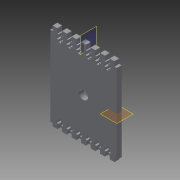
# Autodesk Inventor part: yokeEndBlock
Saved by Autodesk Inventor 2013 (Build 170138000, 138)
## iProperties
Created: 2013-02-24
Part Number: yokeEndBlock
Material: Generic
Document SubType Name: Modeling
Designer: Nano
Density: 1 g/cm^3
d0: 0.250 in
d1: 0.00 deg
d2: 0.250 in
d3: 4.000 ul
d5: 0.500 in
d10: 0.250 in
d11: 0.00 deg
d14: 0.375 in
d21: 0.125 in
d22: 0.600 in
d23: 0.313 in
d24: 0.125 in
d25: 0.375 in
d27: 0.00 deg
d28: 6.000 ul
d30: 0.500 in
Author: Nano
Autodesk Inventor part; units mm, degrees
ref_plane "YZ Plane" through (0, 0, 0) normal (1, 0, 0) x (0, 1, 0)
ref_plane "XZ Plane" through (0, 0, 0) normal (0, 1, 0) x (-1, 0, 0)
ref_plane "XY Plane" through (0, 0, 0) normal (0, 0, 1) x (1, 0, 0)
ref_plane "Work Plane1" through (0, 0, 0) normal (0, 0, 1) x (1, 0, 0)
sketch "Sketch1" plane through (0, 0, 0) normal (0, 0, 1) x (1, 0, 0)
  circle A0 centre (44.45, -59.5313) radius 5.9531
  line L0 (0, 0) -> (0, -116.6812)
  line L1 (0, -116.6812) -> (88.9, -116.6812)
  line L2 (88.9, 0) -> (88.9, -116.6812)
  line L3 (0, 0) -> (88.9, 0)
  dimension "d31" = 11.9062
  dimension "d33" = 116.6813
  constraints: 8 end point, 1 centre point, 1 other
  measures "d31" diameter of A0
  measures "d33" distance of L2.start L1.end
extrude "Extrusion1" add sketch "Sketch1" along normal blind 6.35
sketch "Sketch2" plane through (0, 0, 0) normal (0, 1, 0) x (1, 0, 0)
  line L0 (88.9, 0) -> (0, 0) projected
  line L1 (0, 0) -> (0, -6.35) projected
  line L2 (88.9, -6.35) -> (0, -6.35) projected
  line L3 (88.9, 0) -> (88.9, -6.35) projected
  line L4 (41.275, -6.35) -> (41.275, 0)
  line L5 (41.275, 0) -> (47.625, 0)
  line L6 (47.625, 0) -> (47.625, -6.35)
  line L7 (47.625, -6.35) -> (41.275, -6.35)
  line L8 (41.275, -6.35) -> (47.625, 0) construction
  line L9 (41.275, 0) -> (47.625, -6.35) construction
  line L10 (28.575, -6.35) -> (28.575, 0)
  line L11 (28.575, 0) -> (34.925, 0)
  line L12 (34.925, 0) -> (34.925, -6.35)
  line L13 (34.925, -6.35) -> (28.575, -6.35)
  line L14 (28.575, -6.35) -> (34.925, 0) construction
  line L15 (28.575, 0) -> (34.925, -6.35) construction
  line L16 (15.875, -6.35) -> (15.875, 0)
  line L17 (15.875, 0) -> (22.225, 0)
  line L18 (22.225, 0) -> (22.225, -6.35)
  line L19 (22.225, -6.35) -> (15.875, -6.35)
  line L20 (15.875, -6.35) -> (22.225, 0) construction
  line L21 (15.875, 0) -> (22.225, -6.35) construction
  line L22 (3.175, -6.35) -> (3.175, 0)
  line L23 (3.175, 0) -> (9.525, 0)
  line L24 (9.525, 0) -> (9.525, -6.35)
  line L25 (9.525, -6.35) -> (3.175, -6.35)
  line L26 (3.175, -6.35) -> (9.525, 0) construction
  line L27 (3.175, 0) -> (9.525, -6.35) construction
  line L28 (44.45, 0) -> (44.45, -6.35) construction
  line L29 (60.325, -6.35) -> (60.325, 0)
  line L30 (60.325, 0) -> (53.975, 0)
  line L31 (53.975, 0) -> (53.975, -6.35)
  line L32 (53.975, -6.35) -> (60.325, -6.35)
  line L33 (60.325, -6.35) -> (53.975, 0) construction
  line L34 (60.325, 0) -> (53.975, -6.35) construction
  line L35 (73.025, -6.35) -> (73.025, 0)
  line L36 (73.025, 0) -> (66.675, 0)
  line L37 (66.675, 0) -> (66.675, -6.35)
  line L38 (66.675, -6.35) -> (73.025, -6.35)
  line L39 (73.025, -6.35) -> (66.675, 0) construction
  line L40 (73.025, 0) -> (66.675, -6.35) construction
  line L41 (85.725, -6.35) -> (85.725, 0)
  line L42 (85.725, 0) -> (79.375, 0)
  line L43 (79.375, 0) -> (79.375, -6.35)
  line L44 (79.375, -6.35) -> (85.725, -6.35)
  line L45 (85.725, -6.35) -> (79.375, 0) construction
  line L46 (85.725, 0) -> (79.375, -6.35) construction
  point P0 (44.45, -3.175)
  point P1 (31.75, -3.175)
  point P2 (19.05, -3.175)
  point P3 (6.35, -3.175)
  point P4 (57.15, -3.175)
  point P5 (69.85, -3.175)
  point P6 (82.55, -3.175)
  dimension "d2" = 6.35
  dimension "d5" = 12.7
  constraints: 86 end point, 15 symmetric about line, 14 midpoint, 2 parallel, 1 horizontal, 1 perpendicular, 33 other
  measures "d2" distance of L4.end L5.end
  measures "d5" distance of L4.start L10.start
extrude "Extrusion2" cut sketch "Sketch2" against normal blind 6.35 contours L3 L2 L41 L0 | L43 L2 L35 L0 | L37 L2 L29 L0 | L31 L2 L6 L0 | L4 L2 L12 L0 | L10 L2 L18 L0 | L16 L2 L24 L0 | L22 L2 L1 L0
sketch "Sketch3" plane through (0, 0, 6.35) normal (0, 0, 1) x (1, 0, 0)
  line L0 (47.625, -6.35) -> (47.625, 0) projected
  line L1 (47.625, 0) -> (41.275, 0) projected
  line L2 (41.275, 0) -> (41.275, -6.35) projected
  line L3 (41.275, -6.35) -> (34.925, -6.35) projected
  line L4 (34.925, -6.35) -> (34.925, 0) projected
  line L5 (34.925, 0) -> (28.575, 0) projected
  line L6 (28.575, 0) -> (28.575, -6.35) projected
  line L7 (28.575, -6.35) -> (22.225, -6.35) projected
  line L8 (22.225, -6.35) -> (22.225, 0) projected
  line L9 (22.225, 0) -> (15.875, 0) projected
  line L10 (15.875, 0) -> (15.875, -6.35) projected
  line L11 (15.875, -6.35) -> (9.525, -6.35) projected
  line L12 (9.525, -6.35) -> (9.525, 0) projected
  line L13 (9.525, 0) -> (3.175, 0) projected
  line L14 (3.175, 0) -> (3.175, -6.35) projected
  line L15 (3.175, -6.35) -> (0, -6.35) projected
  line L16 (0, -6.35) -> (0, -116.6813) projected
  line L17 (0, -116.6813) -> (88.9, -116.6813) projected
  line L18 (88.9, -116.6813) -> (88.9, -6.35) projected
  line L19 (88.9, -6.35) -> (85.725, -6.35) projected
  line L20 (85.725, -6.35) -> (85.725, 0) projected
  line L21 (85.725, 0) -> (79.375, 0) projected
  line L22 (79.375, 0) -> (79.375, -6.35) projected
  line L23 (79.375, -6.35) -> (73.025, -6.35) projected
  line L24 (73.025, -6.35) -> (73.025, 0) projected
  line L25 (73.025, 0) -> (66.675, 0) projected
  line L26 (66.675, 0) -> (66.675, -6.35) projected
  line L27 (66.675, -6.35) -> (60.325, -6.35) projected
  line L28 (60.325, -6.35) -> (60.325, 0) projected
  line L29 (60.325, 0) -> (53.975, 0) projected
  line L30 (53.975, 0) -> (53.975, -6.35) projected
  line L31 (53.975, -6.35) -> (47.625, -6.35) projected
  circle A0 centre (44.45, -59.5313) radius 5.9531 projected
  line L32 (0, -59.5313) -> (88.9, -59.5313) construction
  point P0 (0, 0)
  constraints: 2 end point
ref_plane "Work Plane2" through (88.9, -59.5313, 6.35) normal (0, 1, 0) x (-1, 0, 0)
mirror "Mirror1" about plane through (88.9, -59.5313, 6.35) normal (0, 1, 0) of "Extrusion2"
sketch "number6_tSlot01" plane through (0, 0, 6.35) normal (0, 0, 1) x (1, 0, 0)
  line L0 (11.1125, -15.24) -> (14.2875, -15.24)
  line L1 (14.2875, 0) -> (11.1125, 0)
  line L2 (11.1125, -15.24) -> (14.2875, 0) construction
  line L3 (14.2875, -15.24) -> (11.1125, 0) construction
  line L4 (16.6687, -9.1281) -> (16.6687, -12.3031)
  line L5 (8.7312, -12.3031) -> (8.7312, -9.1281)
  line L6 (8.7312, -9.1281) -> (16.6687, -12.3031) construction
  line L7 (16.6687, -9.1281) -> (8.7312, -12.3031) construction
  line L8 (22.225, 0) -> (15.875, 0) projected
  line L9 (8.7312, -9.1281) -> (11.1125, -9.1281)
  line L10 (14.2875, -9.1281) -> (16.6687, -9.1281)
  line L11 (14.2875, -15.24) -> (14.2875, -12.3031)
  line L12 (14.2875, -9.1281) -> (14.2875, 0)
  line L13 (16.6687, -12.3031) -> (14.2875, -12.3031)
  line L14 (11.1125, -12.3031) -> (8.7312, -12.3031)
  line L15 (11.1125, 0) -> (11.1125, -9.1281)
  line L16 (11.1125, -12.3031) -> (11.1125, -15.24)
  point P0 (0, 0)
  point P1 (12.7, -7.62)
  point P2 (12.7, -10.7156)
  dimension "d21" = 3.175
  dimension "d22" = 15.24
  dimension "d23" = 7.9375
  dimension "d24" = 3.175
  constraints: 32 end point, 10 parallel, 4 collinear, 4 midpoint, 4 perpendicular, 3 horizontal, 1 other
  measures "d21" distance of L1.end L1.start
  measures "d22" distance of L1.start L0.end
  measures "d23" distance of L4.end L5.start
  measures "d24" distance of L4.start L4.end
extrude "Extrusion3" cut sketch "number6_tSlot01" against normal through all
pattern_linear "Rectangular Pattern1" count 6 spacing 12.7 along (1, 0, 0) of "Extrusion3"
mirror "Mirror2" about plane through (88.9, -59.5313, 6.35) normal (0, 1, 0) of "Extrusion3", "Rectangular Pattern1"
ref_plane "Work Plane3" through (44.45, 0, 0) normal (-1, 0, 0) x (0, -1, 0)
body "Solid1"
